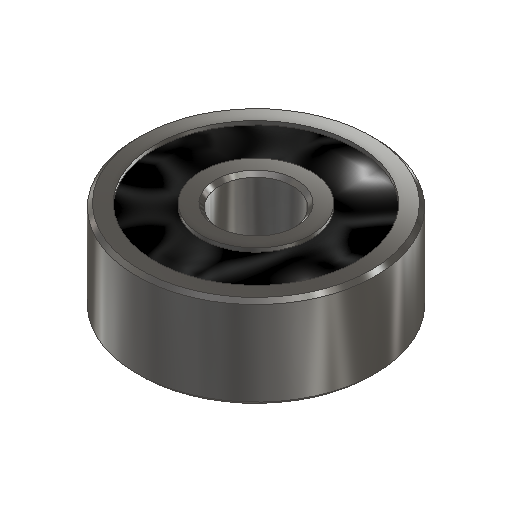
# Autodesk Inventor part: COTS_GENERIC_Bearing_13x4x5
Saved by Autodesk Inventor 2026.1 (Build 301233000, 233)
## iProperties
Created: 2017-05-29
Part Number: COTS_GENERIC_Bearing_13x4x5
Material: Ogólny
Document SubType Name: Modeling
Designer: Andrzej
Density: 1 g/cm^3
Appearance: Stal - polerowana
Mass: 0.57199 g
Surface Area: 5.16216 cm^2
Volume: 0.57199 cm^3
Author: Andrzej
Autodesk Inventor part; units mm, degrees
ref_plane "YZ Plane" through (0, 0, 0) normal (1, 0, 0) x (0, 1, 0)
ref_plane "XZ Plane" through (0, 0, 0) normal (0, 1, 0) x (-1, 0, 0)
ref_plane "XY Plane" through (0, 0, 0) normal (0, 0, 1) x (1, 0, 0)
sketch "Szkic1" plane through (0, 0, 0) normal (0, 0, 1) x (1, 0, 0)
  circle A0 centre (0, 0) radius 6.5
  circle A1 centre (0, 0) radius 2
  dimension "d0" = 13
  dimension "d1" = 4
  constraints: 2 centre point, 2 coincident
  measures "d0" diameter of A0
  measures "d1" diameter of A1
extrude "Wyciągnięcie proste1" add sketch "Szkic1" along normal blind 5
chamfer "Faza1" distance 0.2 angle 45 4 edges at (-2, 0, 5) (-6.5, 0, 5) (-6.5, 0, 0) (-2, 0, 0)
sketch "Szkic2" plane through (0, 0, 5) normal (0, 0, 1) x (1, 0, 0)
  circle A0 centre (0, 0) radius 6.5 projected
  circle A1 centre (0, 0) radius 2 projected
  circle A2 centre (0, 0) radius 5.5
  circle A3 centre (0, 0) radius 3
  dimension "d7" = 1
  dimension "d8" = 1
  constraints: 2 centre point
  measures "d7" radial gap between concentric circles of A0 A2
  measures "d8" radial gap between concentric circles of A1 A3
extrude "Wyciągnięcie proste2" cut sketch "Szkic2" against normal blind 0.2 contours A2
sketch "Szkic3" plane through (0, 0, 0) normal (0, 0, -1) x (-1, 0, 0)
  circle A0 centre (0, 0) radius 5.5 projected
  circle A1 centre (0, 0) radius 6.3 projected
  circle A2 centre (0, 0) radius 2.2 projected
  circle A3 centre (0, 0) radius 3 projected
extrude "Wyciągnięcie proste3" cut sketch "Szkic3" against normal blind 0.2 contours A0
